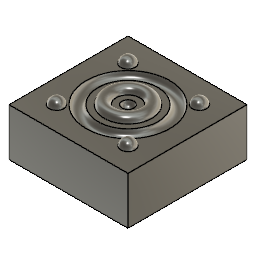
CNC-Machine (Autodesk Fusion 360 design; units mm, degrees)
Autodesk Fusion 360 part; units mm, degrees
sketch "Sketch1" plane through (0, 0, 0) normal (0, 0, 1) x (1, 0, 0)
  line L0 (50, 50) -> (-50, 50)
  line L1 (-50, 50) -> (-50, -50)
  line L2 (-50, -50) -> (50, -50)
  line L3 (50, -50) -> (50, 50)
  line L4 (50, 50) -> (-50, -50) construction
  line L5 (-50, 50) -> (50, -50) construction
  dimension "d1" = 100
  dimension "d2" = 100
  constraint horizontal L0
  constraint perpendicular L0 L1
  constraint parallel L0 L2
  constraint parallel L1 L3
  constraint coincident L4 origin
  constraint coincident L5 origin
  measures "d1" distance of L1.end L2.end
  measures "d2" distance of L0.end L1.end
extrude "Extrude1" add sketch "Sketch1" along normal blind 40
sphere "SpherePrimitive1" cut diameter 10 placed x (-1, 0, 0) y (0, -1, 0) z (0, 0, 1) at (0, 0, 40)
sketch "Sketch3" plane through (0, 0, 40) normal (0, 0, 1) x (-1, 0, 0)
  circle A0 centre (0, 0) radius 5
  line L0 (-50, 50) -> (-50, -50)
  line L1 (-50, -50) -> (50, -50)
  line L2 (50, -50) -> (50, 50)
  line L3 (50, 50) -> (-50, 50)
  line L4 (50, 50) -> (-50, -50) construction
  line L5 (50, -50) -> (-50, 50) construction
  line L6 (-50, 0) -> (50, 0) construction
  line L7 (0, 50) -> (0, -50) construction
  constraint coincident L2.end L3.start
  constraint coincident L0.end L1.start
  constraint coincident L1.end L2.start
  constraint coincident L0.start L3.end
  constraint midpoint L0 L6.start
  constraint midpoint L2 L6.end
  constraint midpoint L3 L7.start
  constraint perpendicular L3 L7
sphere "SpherePrimitive2" add diameter 20 placed x (-1, 0, 0) y (0, -1, 0) z (0, 0, 1) at (-25, -25, 40)
sphere "SpherePrimitive3" add diameter 20 placed x (-1, 0, 0) y (0, -1, 0) z (0, 0, 1) at (25, 25, 40)
torus "TorusPrimitive1" add centre line diameter 30 section diameter 10 placed x (-1, 0, 0) y (0, -1, 0) z (0, 0, 1) at (0, 0, 40)
delete_face "DeleteFace1" 1 faces at (18.3579, 17.6394, 41.3053)
delete_face "DeleteFace2" 1 faces at (-31.6421, -32.3606, 41.3053)
torus "TorusPrimitive2" cut centre line diameter 60 section diameter 10 placed x (-1, 0, 0) y (0, -1, 0) z (0, 0, 1) at (0, 0, 40)
sphere "SpherePrimitive4" add diameter 15 placed x (-1, 0, 0) y (0, -1, 0) z (0, 0, 1) at (40, 40, 40)
sphere "SpherePrimitive5" add diameter 15 placed x (-1, 0, 0) y (0, -1, 0) z (0, 0, 1) at (-40, 40, 40)
sphere "SpherePrimitive6" add diameter 15 placed x (-1, 0, 0) y (0, -1, 0) z (0, 0, 1) at (-40, -40, 40)
sphere "SpherePrimitive7" add diameter 15 placed x (-1, 0, 0) y (0, -1, 0) z (0, 0, 1) at (40, -40, 40)
delete_face "DeleteFace3" 1 faces at (35.0184, 34.4795, 40.9789)
delete_face "DeleteFace4" 1 faces at (-44.9816, 34.4795, 40.9789)
delete_face "DeleteFace5" 1 faces at (-44.9816, -45.5205, 40.9789)
delete_face "DeleteFace6" 1 faces at (35.0184, -45.5205, 40.9789)
sphere "SpherePrimitive8" add diameter 12 placed x (-1, 0, 0) y (0, -1, 0) z (0, 0, 1) at (-30, -30, 40)
sphere "SpherePrimitive9" add diameter 12 placed x (-1, 0, 0) y (0, -1, 0) z (0, 0, 1) at (-30, 30, 40)
sphere "SpherePrimitive10" add diameter 12 placed x (-1, 0, 0) y (0, -1, 0) z (0, 0, 1) at (30, -30, 40)
sphere "SpherePrimitive11" add diameter 12 placed x (-1, 0, 0) y (0, -1, 0) z (0, 0, 1) at (30, 30, 40)
